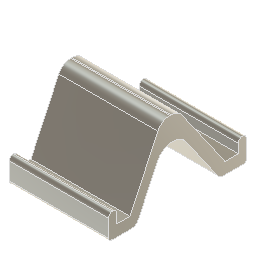
Подставка под телефон (Autodesk Fusion 360 design; units mm, degrees)
Autodesk Fusion 360 part; units mm, degrees
note: some values were not read from the file. Set by a fixed rule: which sketch regions a step uses.
sketch "Sketch1" plane through (0, 0, 0) normal (1, 0, 0) x (0, 1, 0)
  line L0 (0, 0) -> (8, 0)
  line L1 (8, 0) -> (24.8639, 36.1648)
  line L2 (0, 0) -> (0, 8)
  line L3 (0, 8) -> (-5, 8)
  line L4 (-5, 8) -> (-5, -7)
  line L5 (-5, -7) -> (11.814, -7)
  line L6 (11.814, -7) -> (31.9987, 36.2863)
  line L7 (32.1144, 40.7839) -> (32.8533, 40.7839)
  line L8 (39.4065, 37.3725) -> (65.575, 0)
  line L9 (37.0178, 40.7839) -> (86.8057, 40.7839) construction
  line L10 (65.575, 0) -> (73.575, 0)
  line L11 (73.575, 0) -> (73.575, 8)
  line L12 (73.575, 8) -> (78.575, 8)
  line L13 (78.575, 8) -> (78.575, -7)
  line L14 (78.575, -7) -> (62.3081, -7)
  line L15 (31.9987, 36.2863) -> (62.3081, -7)
  line L16 (35, 32) -> (86.0392, 32) construction
  arc A0 (32.1144, 40.7839) -> (24.8639, 36.1648) centre (32.1144, 32.7839) ccw
  arc A1 (39.4065, 37.3725) -> (32.8533, 40.7839) centre (32.8533, 32.7839) ccw
  point P0 (27.0178, 40.7839)
  dimension "d6" = 115
  dimension "d8" = 115
  dimension "d9" = 10
  dimension "d10" = 55
  dimension "d11" = 8
  dimension "d12" = 5
  dimension "d13" = 8
  dimension "d14" = 0
  dimension "d15" = 7
  dimension "d17" = 55
  dimension "d20" = 8
  constraint coincident L0.start L2.start
  constraint horizontal L0
  constraint perpendicular L0 L2
  constraint perpendicular L2 L3
  constraint perpendicular L3 L4
  constraint perpendicular L4 L5
  constraint horizontal L7
  constraint horizontal L9
  constraint parallel L0 L10
  constraint perpendicular L10 L11
  constraint perpendicular L11 L12
  constraint perpendicular L12 L13
  constraint perpendicular L13 L14
  constraint horizontal L16
  constraint coincident P0 L7
  constraint coincident P0 L1
  constraint tangent L7 A0
  constraint tangent L1 A0
  constraint coincident L9.start L7
  constraint coincident L9.start L8
  constraint tangent L7 A1
  constraint tangent L8 A1
  constraint equal A0 A1
  constraint coincident L16.start L15
  measures "d6" angle of L0 L1
  measures "d8" angle of L5 L6
  measures "d9" distance of P0 L9.start
  measures "d10" angle of L8 L9
  measures "d11" distance of L8.end L10.end
  measures "d12" distance of L11.end L12.end
  measures "d13" distance of L10.end L11.end
  measures "d14" distance of L0 L10
  measures "d15" distance of L5 L10
  measures "d17" angle of L15 L16
  measures "d20" radius of A0
extrude "Extrude1" add sketch "Sketch1" along normal blind 60
fillet "Fillet1" radius 2.5 4 edges at (30, 0, 8) (30, -5, 8) (30, 73.575, 8) (30, 78.575, 8)
fillet "Fillet2" radius 10 1 edges at (30, 31.9987, 36.2863)
fillet "Fillet3" radius 5 2 edges at (30, 11.814, -7) (30, 62.3081, -7)
fillet "Fillet4" radius 2 2 edges at (30, -5, -7) (30, 78.575, -7)
